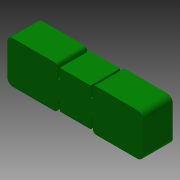
# Autodesk Inventor part: ConnectorDE
Saved by Autodesk Inventor 2015 (Build 190159000, 159)
## iProperties
Created: 2018-01-03
Part Number: ConnectorDE
Material: ABS Plastic
Document SubType Name: Modeling
Designer: Administrator
Density: 1.06 g/cm^3
Appearance: Dark Green
Mass: 13.5173 g
Surface Area: 43.6756 cm^2
Volume: 12.7521 cm^3
Author: Administrator
Autodesk Inventor part; units mm, degrees
ref_plane "YZ Plane" through (0, 0, 0) normal (1, 0, 0) x (0, 1, 0)
ref_plane "XZ Plane" through (0, 0, 0) normal (0, 1, 0) x (-1, 0, 0)
ref_plane "XY Plane" through (0, 0, 0) normal (0, 0, 1) x (1, 0, 0)
sketch "Sketch1" plane through (0, 0, 0) normal (0, 0, 1) x (1, 0, 0)
  line L0 (0, 8.128) -> (-6.604, 8.128)
  line L1 (-6.604, 8.128) -> (-6.604, 3.4598)
  arc A0 (-7.62, 4.4758) -> (-6.604, 3.4598) centre (-6.604, 4.4758) ccw
  line L2 (-7.62, 4.4758) -> (-7.62, 7.779)
  line L3 (-29.21, 6.5078) -> (-29.21, 0)
  arc A1 (-7.62, 7.779) -> (-8.945, 9.0478) centre (-8.89, 7.779) ccw
  line L4 (-8.945, 9.0478) -> (-26.67, 9.0478)
  arc A2 (-26.67, 9.0478) -> (-29.21, 6.5078) centre (-26.67, 6.5078) ccw
  line L5 (0, 8.128) -> (6.604, 8.128)
  line L6 (6.604, 8.128) -> (6.604, 3.4598)
  arc A3 (6.604, 3.4598) -> (7.62, 4.4758) centre (6.604, 4.4758) ccw
  line L7 (7.62, 4.4758) -> (7.62, 7.779)
  line L8 (29.21, 6.5078) -> (29.21, 0)
  arc A4 (8.945, 9.0478) -> (7.62, 7.779) centre (8.89, 7.779) ccw
  line L9 (8.945, 9.0478) -> (26.67, 9.0478)
  arc A5 (29.21, 6.5078) -> (26.67, 9.0478) centre (26.67, 6.5078) ccw
  line L10 (0, -8.128) -> (-6.604, -8.128)
  line L11 (-6.604, -8.128) -> (-6.604, -3.4598)
  arc A6 (-6.604, -3.4598) -> (-7.62, -4.4758) centre (-6.604, -4.4758) ccw
  line L12 (-7.62, -4.4758) -> (-7.62, -7.779)
  line L13 (-29.21, -6.5078) -> (-29.21, 0)
  arc A7 (-8.945, -9.0478) -> (-7.62, -7.779) centre (-8.89, -7.779) ccw
  line L14 (-8.945, -9.0478) -> (-26.67, -9.0478)
  arc A8 (-29.21, -6.5078) -> (-26.67, -9.0478) centre (-26.67, -6.5078) ccw
  line L15 (0, -8.128) -> (6.604, -8.128)
  line L16 (6.604, -8.128) -> (6.604, -3.4598)
  arc A9 (7.62, -4.4758) -> (6.604, -3.4598) centre (6.604, -4.4758) ccw
  line L17 (7.62, -4.4758) -> (7.62, -7.779)
  line L18 (29.21, -6.5078) -> (29.21, 0)
  arc A10 (7.62, -7.779) -> (8.945, -9.0478) centre (8.89, -7.779) ccw
  line L19 (8.945, -9.0478) -> (26.67, -9.0478)
  arc A11 (26.67, -9.0478) -> (29.21, -6.5078) centre (26.67, -6.5078) ccw
  point P0 (0, 0)
  dimension "d0" = 8.128
  dimension "d2" = 29.21
  dimension "d4" = 1.016
  dimension "d5" = 1.016
  dimension "d10" = 1.27
  dimension "d11" = 2.54
  dimension "d12" = 5.588
  constraints: 40 end point, 24 point on circle, 12 centre point, 4 tangent, 2 vertical, 1 horizontal, 1 perpendicular
  measures "d0" distance of point (0, 0) L0.start
  measures "d2" distance of L3.end point (0, 0)
  measures "d4" radius of A0
  measures "d5" distance between parallel lines of L1 L2
  measures "d10" radius of A1
  measures "d11" radius of A2
  measures "d12" distance from line of L1.end L4
extrude "Extrusion1" add sketch "Sketch1" along normal blind 12.7
body "Solid1"
